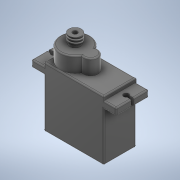
# Autodesk Inventor part: motor servo
Saved by Autodesk Inventor 2020 (Build 240168000, 168)
## iProperties
Created: 2022-09-20
Part Number: motor servo
Material: Generic
Document SubType Name: Modeling
Designer: Dyah Cahya Lestari
Density: 1 g/cm^3
Appearance: Smooth - Black
Author: Dyah Cahya Lestari
Autodesk Inventor part; units mm, degrees
ref_plane "YZ Plane" through (0, 0, 0) normal (1, 0, 0) x (0, 1, 0)
ref_plane "XZ Plane" through (0, 0, 0) normal (0, 1, 0) x (-1, 0, 0)
ref_plane "XY Plane" through (0, 0, 0) normal (0, 0, 1) x (1, 0, 0)
sketch "Sketch1" plane through (0, 0, 0) normal (0, 0, 1) x (1, 0, 0)
  line L0 (0, 0) -> (22.7, 0)
  line L1 (22.7, 0) -> (22.7, -22.7)
  line L2 (22.7, -22.7) -> (0, -22.7)
  line L3 (0, -22.7) -> (0, 0)
  line L4 (22.7, -1.5) -> (27.4, -1.5)
  line L5 (27.4, -1.5) -> (27.4, -4.2)
  line L6 (27.4, -4.2) -> (22.7, -4.2)
  line L7 (22.7, -4.2) -> (22.7, -1.5)
  line L8 (11.35, 0) -> (11.35, -4.2)
  line L9 (0, -1.5) -> (-4.7, -1.5)
  line L10 (-4.7, -1.5) -> (-4.7, -4.2)
  line L11 (-4.7, -4.2) -> (0, -4.2)
  dimension "d0" = 22.7
  dimension "d1" = 22.7
  dimension "d2" = 1.5
  dimension "d3" = 4.7
  dimension "d4" = 2.7
  constraints: 24 end point, 4 parallel, 4 symmetric about line, 2 horizontal, 2 perpendicular, 1 midpoint, 1 point on line, 1 vertical
  measures "d0" distance of L1.end L2.end
  measures "d1" distance of L0.end L1.end
  measures "d2" distance between parallel lines of L0 L4
  measures "d3" distance of L4.start L4.end
  measures "d4" distance of L4.end L5.end
extrude "Extrusion1" add sketch "Sketch1" against normal blind 12.3
sketch "Sketch2" plane through (22.7, -1.5, 0) normal (0, 1, 0) x (1, 0, 0)
  line L0 (4.7, 12.3) -> (0, 12.3) projected
  line L1 (4.7, 0) -> (4.7, 12.3) projected
  arc A0 (3.216, 6.65) -> (3.216, 5.65) centre (2.35, 6.15) ccw
  line L2 (4.7, 6.15) -> (4.7, 6.65)
  line L3 (4.7, 6.65) -> (4.7, 5.65)
  line L4 (4.7, 6.65) -> (3.216, 6.65)
  line L5 (4.7, 5.65) -> (3.216, 5.65)
  line L6 (-22.7, 12.3) -> (0, 12.3) projected
  line L7 (-11.35, 12.3) -> (-11.35, 10.5344)
  line L8 (-27.4, 0) -> (-27.4, 12.3)
  arc A1 (-25.916, 5.65) -> (-25.916, 6.65) centre (-25.05, 6.15) ccw
  line L9 (-27.4, 6.65) -> (-25.916, 6.65)
  line L10 (-27.4, 5.65) -> (-25.916, 5.65)
  point P0 (-22.7, 0)
  point P1 (-27.4, 6.15)
  dimension "d7" = 2
  constraints: 16 end point, 8 symmetric about line, 4 point on circle, 4 point on line, 2 centre point, 2 horizontal, 2 midpoint, 1 vertical, 1 other
  measures "d7" diameter of A0
extrude "Extrusion2" cut sketch "Sketch2" against normal blind 12.3
sketch "Sketch3" plane through (0, 0, 0) normal (0, 1, 0) x (1, 0, 0)
  arc A0 (10.7856, 8.7242) -> (10.7856, 3.5758) centre (5.7, 6.15) ccw
  line L0 (0, 0) -> (0, 12.3) projected
  line L1 (22.7, 0) -> (0, 0) projected
  line L2 (0, 0) -> (0, 12.3) projected
  line L3 (0, 6.15) -> (14.4634, 6.15)
  arc A1 (10.7856, 3.5758) -> (10.7856, 8.7242) centre (11.6, 6.15) ccw
  dimension "d12" = 11.4
  dimension "d13" = 5.7
  dimension "d15" = 12.3
  dimension "d16" = 5.4
  dimension "d17" = 14.3
  constraints: 4 point on circle, 2 centre point, 2 end point, 1 midpoint, 1 perpendicular, 1 point on line
  measures "d12" diameter of A0
  measures "d13" distance from line of L0 A0.centre
  measures "d15" distance of L0.start L0.end
  measures "d16" diameter of A1
extrude "Extrusion3" add sketch "Sketch3" along normal blind 5.7
sketch "Sketch4" plane through (0, 5.7, 0) normal (0, 1, 0) x (1, 0, 0)
  line L0 (0, 0) -> (0, 12.3) projected
  line L1 (0, 6.15) -> (16.0594, 6.15)
  arc A0 (10.7856, 8.7242) -> (10.7856, 3.5758) centre (5.7, 6.15) ccw projected
  circle A1 centre (5.7, 6.15) radius 2
  dimension "d20" = 4
  constraints: 2 end point, 1 centre point, 1 coincident, 1 horizontal, 1 midpoint
  measures "d20" diameter of A1
extrude "Extrusion4" add sketch "Sketch4" along normal blind 1
sketch "Sketch5" plane through (5.7, 6.7, -6.15) normal (0, 1, 0) x (1, 0, 0)
  circle A0 centre (0, 0) radius 2 projected
  circle A1 centre (0, 0) radius 2.35
  point P0 (-5.7, -6.15)
  dimension "d23" = 4.7
  constraints: 1 centre point, 1 coincident
  measures "d23" diameter of A1
extrude "Extrusion5" add sketch "Sketch5" along normal blind 2.7 contours A0 | A1
sketch "Sketch6" plane through (5.7, 9.4, -6.15) normal (0, 1, 0) x (1, 0, 0)
  circle A0 centre (0, 0) radius 0.9
  point P0 (-5.7, -6.15)
  dimension "d26" = 1.8
  constraints: 1 centre point
  measures "d26" diameter of A0
extrude "Extrusion6" cut sketch "Sketch6" against normal blind 0.3
sketch "Sketch7" plane through (5.7, 9.1, -6.15) normal (0, 1, 0) x (1, 0, 0)
  circle A0 centre (0, 0) radius 0.75
  point P0 (-5.7, -6.15)
  dimension "d29" = 1.5
  constraints: 1 centre point
  measures "d29" diameter of A0
extrude "Extrusion7" cut sketch "Sketch7" against normal blind 2
thread "Thread1" size "M1.6x0.35" class "6H" standard "ANSI Metric M Profile" full length
thread "Thread2" size "10-24 UNC" class "3A" standard "ANSI Unified Screw Threads" length 2.7
fillet "Fillet1" radius 0.5 37 edges at (27.4, -2.85, 0) (27.4, -2.85, -12.3) (-4.7, -2.85, -12.3) (-4.7, -2.85, 0) (0, 5.7, -6.15) (14.3, 5.7, -6.15) (0, -13.45, -12.3) (22.7, -13.45, -12.3) (0, -13.45, 0) (22.7, -13.45, 0) (11.35, -22.7, -12.3) (0, -22.7, -6.15) (11.35, -22.7, 0) (22.7, -22.7, -6.15) (11.35, 0, -12.3) (11.35, 0, 0) (0, -0.75, 0) (0, -0.75, -12.3) (0, 0, -9.225) (0, 0, -3.075) (22.7, 0, -6.15) (27.4, -1.5, -2.825) (27.4, -1.5, -9.475) (27.4, -4.2, -9.475) (27.4, -4.2, -2.825) (-4.7, -1.5, -2.825) (-4.7, -4.2, -2.825) (-4.7, -1.5, -9.475) (-4.7, -4.2, -9.475) (-2.35, -1.5, -12.3) (-2.35, -4.2, -12.3) (25.05, -4.2, -12.3) (25.05, -1.5, -12.3) (25.05, -1.5, 0) (-2.35, -1.5, 0) (-2.35, -4.2, 0) (25.05, -4.2, 0)
body "Solid1"
